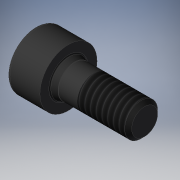
# Autodesk Inventor part: M2.6x66
Saved by Autodesk Inventor 2019 (Build 230136000, 136)
## iProperties
Created: 2023-10-07
Part Number: M2.6x66
Material: Generic
Catalog Web Link: www.cadenas.de
Description: ISO 4762_m26_1-Hexagon Socket Head Cap Screw
Vendor: MISUMI
Document SubType Name: Modeling
Designer: psAdmin
Manufacturer: MISUMI
Mass: 0.0684423 g
Surface Area: 1.22053 cm^2
Volume: 0.0684423 cm^3
Density: 1 g/cm^3
Appearance: PSOLRGB-175-175-175
Category: PARTsolutions
Company: MISUMI
Title: M2.6x66
Author: Cadenas PARTsolutions
Comments: Hexagon Socket Head Cap Screw
PSOL_IDENT_0: {$CADENAS_DATA/23d-libs/misumi/metric/03_set_collars/scsj_m26.prj},164 {VTYP=3D},{NB=M2.6x66},{LINA=
PSOL_IDENT_1: M2.6x66},{NN=ISO 4762_m26_1},{DATE=02.06.2021 02:59:57},{GEOMDATE=20.06.2008 10:25:00},{VERSION=},{L
PSOL_IDENT_2: INEID=2090},{WBVAR=},{WBNUMERIC=}  {NB=M2.6x66},{LINA=M2.6x66},{KT=DUMMY},{D=2.600},{D3=2.048},{P=0.
PSOL_IDENT_3: 450},{L=6.000},{S=2.000},{HM=4.000},{DK=4.500},{DA=3.100},{DS=2.600},{E=2.300},{K=2.600},{R=0.100},{
PSOL_IDENT_4: T=1.100},{V=0.250},{DW=4.180},{W=1.400},{LF=0.510},{LG=1.350},{FORM=1.000},{NENN=M2.6x66}
NB: M2.6x66
NN: ISO 4762_m26_1
NT: Hexagon Socket Head Cap Screw
NBSYN: $NENN.
LINA: M2.6x66
CATALOG: Misumi
D: 2.6
D3: 2.048
P: 0.45
L: 6
S: 2
HM: 4
DK: 4.5
DA: 3.1
DS: 2.6
E: 2.3
K: 2.6
R: 0.1
T: 1.1
V: 0.25
DW: 4.18
W: 1.4
LF: 0.51
LG: 1.35
FORM: 1
SUPPLIER: MISUMI
ARTICLENO: M2.6x66
BOMINFO: M2.6x66
CREATOR: CADENAS GmbH
Autodesk Inventor part; units mm, degrees
sketch "Sketch_1" plane through (0, 0, 0) normal (0, 1, 0) x (-1, 0, 0)
  line L0 (-6, 0) -> (2.61, 0)
  line L1 (0.8226, 0) -> (1.4, -1)
  line L2 (1.4, -1) -> (2.46, -1)
  line L3 (2.46, -1) -> (2.61, -1.15)
  line L4 (2.61, -1.15) -> (2.61, -2)
  arc A0 (2.36, -2.25) -> (2.61, -2) centre (2.36, -2) ccw
  line L5 (2.36, -2.25) -> (0, -2.25)
  line L6 (0, -2.25) -> (0, -1.55)
  arc A1 (0, -1.55) -> (-0.0656, -1.4561) centre (-0.1, -1.55) ccw
  line L7 (-0.0656, -1.4561) -> (-0.4756, -1.3061)
  arc A2 (-0.4756, -1.3061) -> (-0.51, -1.3) centre (-0.51, -1.4) ccw
  line L8 (-0.51, -1.3) -> (-5.724, -1.3)
  line L9 (-5.724, -1.3) -> (-6, -1.024)
  line L10 (-6, -1.024) -> (-6, 0)
  line L11 (-6, 0) -> (0.8226, 0)
  constraints: 24 end point, 6 point on circle, 3 centre point
revolve "Revolution1" add sketch "Sketch_1" angle 360 about axis through (6, 0, 0) along (1, 0, 0)
thread "Thread1" size "M2.6x0.45" class "6g" standard "ISO Metric profile" length 3.724
sketch "Skizze_1" plane through (-1.4, 0, 0) normal (1, 0, 0) x (0, 0, -1)
  line L0 (-1, -0.5774) -> (0, -1.1547)
  line L1 (0, -1.1547) -> (1, -0.5774)
  line L2 (1, -0.5774) -> (1, 0.5774)
  line L3 (1, 0.5774) -> (0, 1.1547)
  line L4 (0, 1.1547) -> (-1, 0.5774)
  line L5 (-1, 0.5774) -> (-1, -0.5774)
  constraints: 12 end point
extrude "Extrusion1" cut sketch "Skizze_1" against normal blind 2.2
ref_plane "IP1_XY" through (0, 0, 0) normal (1, 0, 0) x (0, 0, -1)
ref_plane "IP1_YZ" through (0, 0, 0) normal (0, 0, -1) x (0, 1, 0)
ref_plane "IP1_ZX" through (0, 0, 0) normal (0, 1, 0) x (1, 0, 0)
ref_plane "IP2_XY" through (-2.6, 0, 0) normal (1, 0, 0) x (0, 0, -1)
ref_plane "IP2_YZ" through (-2.6, 0, 0) normal (0, 0, -1) x (0, 1, 0)
ref_plane "IP2_ZX" through (-2.6, 0, 0) normal (0, 1, 0) x (1, 0, 0)
ref_plane "IP3_XY" through (6, 0, 0) normal (1, 0, 0) x (0, 0, -1)
ref_plane "IP3_YZ" through (6, 0, 0) normal (0, 0, -1) x (0, 1, 0)
ref_plane "IP3_ZX" through (6, 0, 0) normal (0, 1, 0) x (1, 0, 0)
ref_plane "IP4_XY" through (0, 0, 0) normal (1, 0, 0) x (0, 0, -1)
ref_plane "IP4_YZ" through (0, 0, 0) normal (0, 0, -1) x (0, 1, 0)
ref_plane "IP4_ZX" through (0, 0, 0) normal (0, 1, 0) x (1, 0, 0)
body "Solid1"
